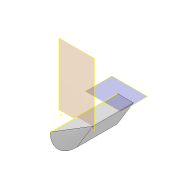
# Autodesk Inventor part: encoder guard
Saved by Autodesk Inventor 2020 (Build 240168000, 168)
## iProperties
Created: 2020-01-15
Part Number: encoder guard
Material: Generic
Document SubType Name: Modeling
Designer: ball
Density: 1 g/cm^3
Appearance: Default
Author: ball
Autodesk Inventor part; units mm, degrees
ref_plane "YZ Plane" through (0, 0, 0) normal (1, 0, 0) x (0, 1, 0)
ref_plane "XZ Plane" through (0, 0, 0) normal (0, 1, 0) x (-1, 0, 0)
ref_plane "XY Plane" through (0, 0, 0) normal (0, 0, 1) x (1, 0, 0)
ref_plane "Work Plane1" through (0, 0, 0) normal (0, 0, 1) x (1, 0, 0)
sketch "Sketch1" plane through (0, 0, 0) normal (0, 0, 1) x (1, 0, 0)
  line L0 (25.4, -44.45) -> (0, -44.45) construction
  line L1 (25.4, -44.45) -> (12.7, -44.45)
  line L2 (12.7, -65.151) -> (25.4, -44.45)
  line L3 (12.7, -44.45) -> (12.7, -65.151)
  point P0 (0, 0)
  dimension "d0" = 20.701
  dimension "d1" = 12.7
  constraints: 6 end point, 1 midpoint, 1 perpendicular, 1 point on line
  measures "d0" distance from line of L0 L2.start
  measures "d1" distance from line of L1.start L3
revolve "Revolution1" add sketch "Sketch1" angle 180 mid plane about axis through (25.4, -44.45, 0) along (-1, 0, 0)
ref_plane "Work Plane2" through (12.7, -44.45, -31.115) normal (0, -1, 0) x (0, 0, -1)
sketch "Sketch2" plane through (12.7, -44.45, -31.115) normal (0, -1, 0) x (0, 0, -1)
  line L0 (0.635, -12.7) -> (0.635, 12.7) construction
  line L1 (9.525, 12.7) -> (-9.525, 12.7) construction
  line L2 (0.635, 0) -> (-31.115, 0)
  line L3 (-31.115, 0) -> (-31.115, 12.7)
  line L4 (-31.115, 12.7) -> (0.635, 12.7)
  line L5 (0.635, 12.7) -> (0.635, 0)
  point P0 (-31.115, -12.7)
  constraints: 8 end point, 2 parallel, 1 horizontal, 1 midpoint, 1 perpendicular
extrude "Extrusion1" add sketch "Sketch2" along normal blind 5.08
sketch "Sketch3" plane through (12.7, -49.53, -31.115) normal (0, -1, 0) x (1, 0, 0)
  point P0 (-12.7, 31.115)
sketch "Sketch4" plane through (25.4, -44.45, -31.75) normal (0, 0, -1) x (-1, 0, 0)
  line L0 (12.7, -5.08) -> (3.1166, -5.08)
  line L1 (0, 0) -> (12.7, -20.701) projected
  line L2 (12.7, -20.701) -> (12.7, 0) projected
  line L3 (12.7, -5.08) -> (12.7, -20.701)
  line L4 (12.7, -20.701) -> (3.1166, -5.08)
  point P0 (25.4, 44.45)
  constraints: 6 end point, 1 collinear, 1 horizontal, 1 point on line
extrude "Extrusion2" add sketch "Sketch4" against normal through all
fillet "Fillet1" radius 1.905 2 edges at (22.2834, -49.53, -15.875) (25.4, -49.53, -15.875)
sketch "Sketch5" plane through (25.4, -47.625, 0) normal (0, 0, 1) x (1, 0, 0)
  line L0 (-12.7, 3.175) -> (0, 3.175) projected
  line L1 (-3.6741, -2.8138) -> (0, 3.175) projected
  line L2 (0, 3.175) -> (-3.6741, -2.8138)
  line L3 (-3.6741, -2.8138) -> (0, -4.7625)
  line L4 (0, -4.7625) -> (4.0347, 1.814)
  line L5 (4.0347, 1.814) -> (0, 3.175)
  point P0 (-25.4, 47.625)
  constraints: 8 end point, 1 collinear, 1 parallel
extrude "Extrusion3" cut sketch "Sketch5" against normal through all
sketch "Sketch6" plane through (12.7, -44.45, 20.701) normal (0, 1, 0) x (1, 0, 0)
  line L0 (0, 0) -> (0, 52.451) projected
  point P0 (-12.7, 20.701)
body "Solid1"
